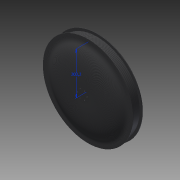
# Autodesk Inventor part: wheel_rim
Saved by Autodesk Inventor 2014 (Build 180170000, 170)
## iProperties
Created: 2014-03-12
Part Number: wheel_rim
Material: PRFC
Document SubType Name: Modeling
Designer: Yann
Density: 1.43 g/cm^3
Appearance: Fibre de carbone
d9: 3,000 mm
d14: 0,00 deg
d_profile_section: 40,000 mm
d_prfc_thickness: 3,000 mm
d_arm_in_diameter: 27,000 mm
d_arm_out_diameter: 30,000 mm
d_arm_length: 250,000 mm
d_suspension_height: 140,000 mm
d_aluminum_thickness: 3,175 mm
d_suspension_box_width: 40,000 mm
d_wheelbase: 1600,000 mm
a_tilt: 10,00 deg
d_rear_profile_height: 101,600 mm
d_rear_profile_width: 50,800 mm
d_central_profile_width: 50,800 mm
d_central_profile_height: 101,600 mm
d_handle_bar_tube_diameter: 35,000 mm
a_direction_column: 35,00 deg
prfc_tube_id: 33,000 mm
prfc_tube_od: 35,000 mm
front_suspension_height: 140,930 mm
front_suspension_width: 150,000 mm
caster_angle: 24,00 deg
a_caster_angle: 25,00 deg
d_handlebar_pivot_offset: 65,000 mm
d_handlebar_arm_length: 80,000 mm
a_handlebar_angle: 60,00 deg
d_left_to_right_front_pivots: 28,000 mm
d_front_arm_id: 29,261 mm
d_front_arm_od: 31,750 mm
d_aluminum_bar_thickness: 12,700 mm
d_handle_bar_id: 30,000 mm
d_handle_bar_od: 38,100 mm
d_steering_arm_length: 70,000 mm
d_steering_height_from_hub_center: 28,000 mm
d_steering_height_from_hub_carrier_center: 18,000 mm
Author: Yann
Autodesk Inventor part; units mm, degrees
ref_plane "YZ Plane" through (0, 0, 0) normal (1, 0, 0) x (0, 1, 0)
ref_plane "XZ Plane" through (0, 0, 0) normal (0, 1, 0) x (-1, 0, 0)
ref_plane "XY Plane" through (0, 0, 0) normal (0, 0, 1) x (1, 0, 0)
sketch "Esquisse1" plane through (0, 0, 0) normal (1, 0, 0) x (0, 1, 0)
  line L0 (0, -56) -> (0, 56)
  line L1 (-49.4, 0) -> (30.4, 0)
  line L2 (-47.5, 32) -> (-47.5, 0)
  line L3 (23.32, 200.2) -> (-20.32, 200.2)
  line L4 (-50.5, 0) -> (-50.5, 32)
  line L5 (-47.5, 0) -> (-50.5, 0)
  line L6 (-50.5, 0) -> (-47.5, 0)
  line L7 (-47.5, 32) -> (-50.5, 32) construction
  line L8 (-47.5, -30) -> (-47.5, 30) projected
  line L9 (-17.32, -203.2) -> (-17.32, 203.2) construction
  line L10 (-20.32, -203.2) -> (-20.32, 203.2) construction
  line L11 (18.32, 203.2) -> (18.32, -203.2) construction
  line L12 (17.32, -203.2) -> (17.32, 203.2) construction
  line L13 (20.32, -203.2) -> (20.32, 203.2) construction
  line L14 (20.32, 215.2) -> (23.32, 215.2)
  line L15 (23.32, 215.2) -> (23.32, 200.2)
  line L16 (-23.32, 200.2) -> (-23.32, 215.2)
  line L17 (-23.32, 215.2) -> (-20.32, 215.2)
  line L18 (-20.32, 215.2) -> (-20.32, 203.2)
  line L19 (-20.32, 203.2) -> (20.32, 203.2)
  line L20 (20.32, 203.2) -> (20.32, 215.2)
  line L21 (-20.32, 200.2) -> (-23.32, 200.2) construction
  line L22 (20.32, 203.2) -> (20.32, 200.2) construction
  line L23 (-20.32, 200.2) -> (-20.32, 180.2) construction
  line L24 (-20.32, 180.2) -> (-33.0773, 176.0923) construction
  line L25 (-33.0773, 176.0923) -> (-50, 129.3731) construction
  line L26 (-50, 129.3731) -> (-47.5, 42) construction
  line L27 (-47.5, 42) -> (-47.5, 32) construction
  spline S0 degree 4 poles (-20.32, 200.2) (-20.32, 180.2) (-33.0773, 176.0923) (-50, 129.3731) (-47.5, 42) (-47.5, 32) knots 1 1 1 1 1 2 3 3 3 3 3
  spline S1 degree 5 poles (-23.32, 200.2) (-23.3199, 198.3844) (-23.3716, 196.5688) (-23.4859, 194.7552) (-23.8349, 191.6186) (-24.5084, 188.5383) (-24.8603, 187.248) (-25.6789, 184.7885) (-26.7147, 182.4126) (-27.2583, 181.281) (-28.4715, 178.8909) (-29.747, 176.5332) (-30.4258, 175.2799) (-31.9037, 172.5044) (-33.3133, 169.6936) (-34.0545, 168.1423) (-35.6303, 164.6693) (-37.0531, 161.1305) (-37.7885, 159.1688) (-39.3183, 154.8027) (-40.6538, 150.3728) (-41.332, 147.9334) (-42.7081, 142.5835) (-43.8774, 137.1842) (-44.457, 134.2482) (-45.5952, 127.9452) (-46.5359, 121.6095) (-46.9881, 118.227) (-47.8405, 111.1566) (-48.5208, 104.0676) (-48.8338, 100.3717) (-49.3914, 92.8899) (-49.8093, 85.3989) (-49.9882, 81.6095) (-50.2781, 74.2453) (-50.4635, 66.8779) (-50.5309, 63.3022) (-50.6147, 56.7606) (-50.6326, 50.2184) (-50.6275, 47.2525) (-50.6011, 42.4224) (-50.5494, 37.5925) (-50.531, 35.7284) (-50.5018, 33.8642) (-50.5, 32) knots 0 0 0 0 0 0 0.052645 0.052645 0.052645 0.091341 0.091341 0.091341 0.127725 0.127725 0.127725 0.169058 0.169058 0.169058 0.218895 0.218895 0.218895 0.27962 0.27962 0.27962 0.353015 0.353015 0.353015 0.439772 0.439772 0.439772 0.538713 0.538713 0.538713 0.646254 0.646254 0.646254 0.75625 0.75625 0.75625 0.859944 0.859944 0.859944 0.945945 0.945945 0.945945 1 1 1 1 1 1
  point P0 (0, 0)
  point P1 (-20.32, 200.2)
  dimension "d9" = 3
  dimension "d16" = 203.2
  dimension "d17" = 12
  dimension "d19" = 32
  dimension "d21" = 20
  dimension "d22" = 10
  constraints: 38 end point, 7 equal length, 7 point on line, 5 horizontal, 4 collinear, 4 vertical, 3 perpendicular, 1 midpoint, 1 parallel, 12 other
  measures "d9" distance between parallel lines of L4 L2
  measures "d16" distance between parallel lines of L1 L19
  measures "d17" distance between parallel lines of L17 L19
  measures "d19" distance between parallel lines of L7 L1
  measures "d21" distance from line of L23.end L21
  measures "d22" distance from line of L26.end L7
revolve "Révolution1" add sketch "Esquisse1" angle 360 about axis through (0, -49.4, 0) along (0, 1, 0)
sketch "Esquisse2" plane through (0, 0, 0) normal (0, 1, 0) x (-1, 0, 0)
  circle A0 centre (11, 19.0526) radius 2.5
  circle A1 centre (-11, 19.0526) radius 2.5
  circle A2 centre (-22, 0) radius 2.5
  circle A3 centre (-11, -19.0526) radius 2.5
  circle A4 centre (11, -19.0526) radius 2.5
  circle A5 centre (22, 0) radius 2.5
  circle A6 centre (-11, -19.0526) radius 2.5
  circle A7 centre (11, -19.0526) radius 2.5
  circle A8 centre (22, 0) radius 2.5
  circle A9 centre (11, 19.0526) radius 2.5
  circle A10 centre (-11, 19.0526) radius 2.5
  circle A11 centre (-22, 0) radius 2.5
  circle A12 centre (0, 0) radius 30
  circle A13 centre (0, 0) radius 13
  point P0 (0, 0)
extrude "Extrusion1" cut sketch "Esquisse2" against normal through all contours A0 | A1 | A2 | A3 | A4 | A5
fillet "Congé1" [suppressed]
fillet "Congé3" radius 7.25 1 edges at (0, -20.32, -200.2)
equation "\"d_profile_section\" = 40"
equation "\"d_prfc_thickness\" = 3"
equation "\"d_arm_in_diameter\" = 27"
equation "\"d_arm_out_diameter\" = 30"
equation "\"d_arm_length\" = 250"
equation "\"d_suspension_height\" = 140"
equation "\"d_aluminum_thickness\" = 3.175"
equation "\"d_suspension_box_width\" = 40"
equation "\"d_wheelbase\" = 1600"
equation "\"a_tilt\" = 10deg"
equation "\"d_rear_profile_height\" = 101.6"
equation "\"d_rear_profile_width\" = 50.8"
equation "\"d_central_profile_width\" = 50.8"
equation "\"d_central_profile_height\" = 101.6"
equation "\"d_handle_bar_tube_diameter\" = 35"
equation "\"a_direction_column\" = 35deg"
equation "\"prfc_tube_id\" = 33"
equation "\"prfc_tube_od\" = 35"
equation "\"front_suspension_height\" = 140.92977"
equation "\"front_suspension_width\" = 150"
equation "\"caster_angle\" = 24deg"
equation "\"a_caster_angle\" = 25deg"
equation "\"d_handlebar_pivot_offset\" = 65"
equation "\"d_handlebar_arm_length\" = 80"
equation "\"a_handlebar_angle\" = 60deg"
equation "\"d_left_to_right_front_pivots\" = 28"
equation "\"d_front_arm_id\" = 29.2608"
equation "\"d_front_arm_od\" = 31.75"
equation "\"d_aluminum_bar_thickness\" = 12.7"
equation "\"d_handle_bar_id\" = 30"
equation "\"d_handle_bar_od\" = 38.1"
equation "\"d_steering_arm_length\" = 70"
equation "\"d_steering_height_from_hub_center\" = 28"
equation "\"d_steering_height_from_hub_carrier_center\" = 18"
equation "\"d_central_beam_inclination\" = 12"
equation "\"a_central_beam_inclination\" = 12deg"
equation "\"d_central_beam_screws_diameter\" = 8"
equation "\"d_rear_profile_wall_thickness\" = 4.7625"
equation "\"d_rear_profile_wall_thickness_1\" = 4.7625"
equation "\"d_central_pivot_screw_diameter\" = 15.875"
